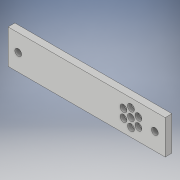
# Autodesk Inventor part: core hex motor to 30x30 mount
Saved by Autodesk Inventor 2019 (Build 230136000, 136)
## iProperties
Created: 2017-12-08
Part Number: core hex motor to 30x30 mount
Material: Generic
Document SubType Name: Modeling
Designer: User
Density: 1 g/cm^3
Appearance: Default
Author: User
Autodesk Inventor part; units mm, degrees
ref_plane "YZ Plane" through (0, 0, 0) normal (1, 0, 0) x (0, 1, 0)
ref_plane "XZ Plane" through (0, 0, 0) normal (0, 1, 0) x (-1, 0, 0)
ref_plane "XY Plane" through (0, 0, 0) normal (0, 0, 1) x (1, 0, 0)
sketch "Sketch1" plane through (0, 0, 0) normal (0, 0, 1) x (1, 0, 0)
  line L0 (0, 0) -> (146.05, 0)
  line L1 (146.05, 0) -> (146.05, 31.75)
  line L2 (146.05, 31.75) -> (0, 31.75)
  line L3 (0, 31.75) -> (0, 0)
  dimension "d0" = 146.05
  dimension "d1" = 31.75
  constraints: 8 end point, 2 parallel, 1 horizontal, 1 perpendicular
  measures "d0" distance of L2.end L1.end
  measures "d1" distance of L1.end L0.end
extrude "Extrusion1" add sketch "Sketch1" along normal blind 6.35
sketch "Sketch2" plane through (0, 0, 6.35) normal (0, 0, 1) x (1, 0, 0)
  line L0 (146.05, 0) -> (146.05, 31.75) projected
  line L1 (146.05, 12.7901) -> (163.1696, 12.7901) construction
  line L2 (0, 0) -> (146.05, 0) projected
  line L3 (114.3, 0) -> (114.3, 15.875)
  line L4 (114.3, 0) -> (130.175, 0) construction
  circle A0 centre (114.3, 15.875) radius 8.001
  point P0 (114.3, 7.874)
  point P1 (121.2291, 11.8745)
  point P2 (121.2291, 19.8755)
  point P3 (114.3, 23.876)
  point P4 (107.3709, 19.8755)
  point P5 (107.3709, 11.8745)
  dimension "d9" = 16.002
  dimension "d7" = 90
  dimension "d17" = 31.75
  dimension "d48" = 360
  dimension "d79" = 31.75
  dimension "d80" = 15.875
  dimension "d81" = 15.875
  constraints: 6 end point, 3 point on line, 2 horizontal, 2 perpendicular, 1 coincident, 1 vertical alignment, 9 other
  measures "d7" angle of L4 L3
  measures "d17" distance from line of L0 L3.end
  measures "d79" distance of L0.start L0.end
  measures "d80" distance from line of L2 point (114.3, 15.875)
  measures "d81" distance from line of L2 L3.end
hole "Hole2" at (114.3, 7.874, 6.35) at (121.2291, 11.8745, 6.35) at (121.2291, 19.8755, 6.35) at (114.3, 23.876, 6.35) at (107.3709, 19.8755, 6.35) at (107.3709, 11.8745, 6.35) direction (0, 0, -1) diameter 3.4036 end through all counterbore diameter 6.5024 counterbore depth 3.4036 clearance for "Socket Head Cap Screw ISO 4762" size "M3" standard "ISO"
hole "Hole3" at (114.3, 15.875, 6.35) direction (0, 0, -1) diameter 6.35 end through all
sketch "Sketch5" plane through (0, 0, 6.35) normal (0, 0, 1) x (1, 0, 0)
  line L0 (0, 31.75) -> (0, 0) projected
  line L1 (146.05, 31.75) -> (0, 31.75) projected
  circle A0 centre (114.3, 15.875) radius 3.175 projected
  circle A1 centre (107.3709, 19.8755) radius 3.2512 projected
  circle A2 centre (121.2291, 19.8755) radius 3.2512 projected
  circle A3 centre (114.3, 7.874) radius 3.2512 projected
  circle A4 centre (121.2291, 11.8745) radius 3.2512 projected
  circle A5 centre (114.3, 23.876) radius 3.2512 projected
  circle A6 centre (107.3709, 11.8745) radius 3.2512 projected
  line L2 (0, 0) -> (146.05, 0) projected
  line L3 (146.05, 0) -> (146.05, 31.75) projected
  line L4 (146.05, 31.75) -> (0, 31.75) projected
  line L5 (0, 31.75) -> (0, 0) projected
  point P0 (9.525, 15.875)
  point P1 (136.525, 15.875)
  dimension "d64" = 31.75
  dimension "d65" = 15.875
  dimension "d68" = 15.875
  dimension "d69" = 9.525
  dimension "d71" = 9.525
  measures "d64" distance of L0.start L0.end
  measures "d65" distance from line of L1 point (9.525, 15.875)
  measures "d68" distance from line of L1 point (136.525, 15.875)
  measures "d69" distance from line of L0 point (9.525, 15.875)
  measures "d71" distance from line of L3 point (136.525, 15.875)
hole "Hole4" at (9.525, 15.875, 6.35) at (136.525, 15.875, 6.35) direction (0, 0, -1) diameter 6.35 end through all
equation "\"d80\" = 0.5 * d79"
equation "\"d81\" = d80"
equation "\"d65\" = 0.5 * d64"
equation "\"d68\" = d65"
equation "\"d69\" = d71"
body "Solid1"
